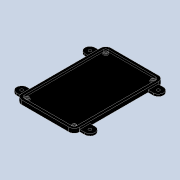
# Autodesk Inventor part: BTT Octopus 1.1 Mount
Saved by Autodesk Inventor 2022 (Build 260153000, 153)
## iProperties
Created: 2022-01-02
Part Number: BTT Octopus 1.1 Mount
Material: Generic
Document SubType Name: Modeling
Designer: Coy
Density: 1 g/cm^3
Appearance: Anodized - Black
Author: Coy
Autodesk Inventor part; units mm, degrees
ref_plane "YZ Plane" through (0, 0, 0) normal (1, 0, 0) x (0, 1, 0)
ref_plane "XZ Plane" through (0, 0, 0) normal (0, 1, 0) x (-1, 0, 0)
ref_plane "XY Plane" through (0, 0, 0) normal (0, 0, 1) x (1, 0, 0)
sketch "Sketch1" plane through (0, 0, 0) normal (0, 1, 0) x (-1, 0, 0)
  line L0 (5, 0) -> (95.5, 0)
  line L1 (100.5, 5) -> (100.5, 155.5)
  line L2 (95.5, 160.5) -> (5, 160.5)
  line L3 (0, 155.5) -> (0, 5)
  arc A0 (100.5, 155.5) -> (95.5, 160.5) centre (95.5, 155.5) ccw
  arc A1 (95.5, 0) -> (100.5, 5) centre (95.5, 5) ccw
  arc A2 (0, 5) -> (5, 0) centre (5, 5) ccw
  arc A3 (5, 160.5) -> (0, 155.5) centre (5, 155.5) ccw
  line L4 (105.5, 155.5) -> (105.5, 5)
  arc A4 (95.5, -5) -> (105.5, 5) centre (95.5, 5) ccw
  line L5 (95.5, -5) -> (5, -5)
  arc A5 (-5, 5) -> (5, -5) centre (5, 5) ccw
  line L6 (-5, 5) -> (-5, 155.5)
  arc A6 (5, 165.5) -> (-5, 155.5) centre (5, 155.5) ccw
  line L7 (5, 165.5) -> (95.5, 165.5)
  arc A7 (105.5, 155.5) -> (95.5, 165.5) centre (95.5, 155.5) ccw
  point P0 (0, 0)
  point P1 (100.5, 160.5)
  point P2 (100.5, 0)
  point P3 (0, 160.5)
  dimension "d0" = 100.5
  dimension "d1" = 160.5
  dimension "d2" = 5
  dimension "d3" = 5
  constraints: 16 end point, 16 point on circle, 8 centre point, 8 point on line, 8 tangent, 4 parallel, 3 equal radius, 2 perpendicular, 1 horizontal, 7 other
  measures "d0" distance of point (0, 160.5) point (100.5, 160.5)
  measures "d1" distance of point (100.5, 160.5) point (100.5, 0)
  measures "d2" radius of A0
  measures "d3" distance between parallel lines of L1 L4
extrude "Extrusion1" add sketch "Sketch1" along normal blind 4
sketch "Sketch2" plane through (0, 0, 0) normal (0, -1, 0) x (1, 0, 0)
  line L0 (5, 155.5) -> (5, 5) projected
  arc A0 (5, 155.5) -> (-5, 165.5) centre (-5, 155.5) ccw projected
  line L1 (-95.5, 165.5) -> (-5, 165.5) projected
  arc A1 (-95.5, 165.5) -> (-105.5, 155.5) centre (-95.5, 155.5) ccw projected
  line L2 (-105.5, 5) -> (-105.5, 155.5) projected
  arc A2 (-105.5, 5) -> (-95.5, -5) centre (-95.5, 5) ccw projected
  line L3 (-5, -5) -> (-95.5, -5) projected
  arc A3 (-5, -5) -> (5, 5) centre (-5, 5) ccw projected
  arc A4 (-5, 0) -> (0, 5) centre (-5, 5) ccw projected
  line L4 (-95.5, 0) -> (-5, 0) projected
  arc A5 (-100.5, 5) -> (-95.5, 0) centre (-95.5, 5) ccw projected
  line L5 (-100.5, 155.5) -> (-100.5, 5) projected
  arc A6 (-95.5, 160.5) -> (-100.5, 155.5) centre (-95.5, 155.5) ccw projected
  line L6 (-5, 160.5) -> (-95.5, 160.5) projected
  arc A7 (0, 155.5) -> (-5, 160.5) centre (-5, 155.5) ccw projected
  line L7 (0, 5) -> (0, 155.5) projected
  line L8 (14.75, 145.25) -> (-115.25, 145.25) construction
  line L9 (-115.25, 145.25) -> (-115.25, 15.25) construction
  line L10 (-115.25, 15.25) -> (14.75, 15.25) construction
  line L11 (14.75, 15.25) -> (14.75, 145.25) construction
  circle A8 centre (14.75, 145.25) radius 2.75
  arc A9 (14.75, 135.5) -> (14.75, 155) centre (14.75, 145.25) ccw
  line L12 (5, 155.5) -> (5, 5) projected
  line L13 (5, 155.5) -> (5, 5) projected
  line L14 (5, 135.5) -> (14.75, 135.5)
  line L15 (5, 155) -> (14.75, 155)
  line L16 (0, 5) -> (0, 155.5) construction
  line L17 (0, 80.25) -> (-100.5, 80.25) construction
  line L18 (-100.5, 155.5) -> (-100.5, 5) construction
  line L19 (-50.25, 80.25) -> (-50.25, 145.25) construction
  circle A10 centre (14.75, 15.25) radius 2.75
  arc A11 (14.75, 5.5) -> (14.75, 25) centre (14.75, 15.25) ccw
  line L20 (5, 25) -> (14.75, 25)
  line L21 (5, 5.5) -> (14.75, 5.5)
  circle A12 centre (-115.25, 145.25) radius 2.75
  arc A13 (-115.25, 155) -> (-115.25, 135.5) centre (-115.25, 145.25) ccw
  line L22 (-105.5, 135.5) -> (-115.25, 135.5)
  line L23 (-105.5, 155) -> (-115.25, 155)
  arc A14 (-115.25, 25) -> (-115.25, 5.5) centre (-115.25, 15.25) ccw
  line L24 (-105.5, 25) -> (-115.25, 25)
  circle A15 centre (-115.25, 15.25) radius 2.75
  line L25 (-105.5, 5.5) -> (-115.25, 5.5)
  point P0 (0, 0)
  dimension "d6" = 130
  dimension "d7" = 130
  dimension "d8" = 110.5
  dimension "d9" = 9.75
  dimension "d10" = 170.5
  dimension "d11" = 20.25
  dimension "d12" = 5.5
  constraints: 28 end point, 15 symmetric about line, 8 centre point, 8 point on circle, 4 midpoint, 3 perpendicular, 3 tangent, 2 parallel, 2 point on line, 1 coincident, 1 horizontal, 6 other
  measures "d6" distance of L10.end L9.end
  measures "d7" distance of L9.end L8.end
  measures "d8" distance between parallel lines of L2 L0
  measures "d9" distance between parallel lines of L0 L11
  measures "d10" distance between parallel lines of L3 L1
  measures "d11" distance between parallel lines of L1 L8
  measures "d12" diameter of A8
extrude "Extrusion2" add sketch "Sketch2" along normal blind 4 contours L0 A3 L3 A2 L2 A1 L1 A0 | L15 A9 L14 L0 | L20 A11 L21 L0 | L2 L22 A13 L23 | L2 L25 A14 L24 | L4 A5 L5 A6 L6 A7 L7 A4
sketch "Sketch3" plane through (0, 0, 0) normal (0, 1, 0) x (1, 0, 0)
  line L0 (-5.25, -155.25) -> (-95.25, -155.25) construction
  line L1 (-95.25, -155.25) -> (-95.25, -5.25) construction
  line L2 (-95.25, -5.25) -> (-5.25, -5.25) construction
  line L3 (-5.25, -5.25) -> (-5.25, -155.25) construction
  line L4 (-50.25, -155.25) -> (-50.25, -160.5) construction
  line L5 (-5, -160.5) -> (-95.5, -160.5) construction
  line L6 (-5.25, -80.25) -> (0, -80.25) construction
  line L7 (-50.25, -5.25) -> (-50.25, 0) construction
  line L8 (-95.5, 0) -> (-5, 0) construction
  line L9 (-95.25, -80.25) -> (-100.5, -80.25) construction
  line L10 (-100.5, -155.5) -> (-100.5, -5) construction
  line L11 (0, -5) -> (0, -155.5) projected
  line L12 (-100.5, -155.5) -> (-100.5, -5) projected
  arc A0 (-5, -160.5) -> (0, -155.5) centre (-5, -155.5) ccw projected
  arc A1 (-100.5, -155.5) -> (-95.5, -160.5) centre (-95.5, -155.5) ccw projected
  circle A2 centre (-5.25, -5.25) radius 3.5
  circle A3 centre (-5.25, -155.25) radius 3.5
  circle A4 centre (-95.25, -155.25) radius 3.5
  circle A5 centre (-95.25, -5.25) radius 3.5
  point P0 (0, 0)
  dimension "d15" = 90
  dimension "d16" = 150
  dimension "d17" = 7
  dimension "d18" = 7
  dimension "d19" = 7
  dimension "d20" = 7
  constraints: 16 end point, 8 midpoint, 4 centre point, 4 coincident, 4 parallel, 2 collinear, 2 horizontal, 2 perpendicular, 2 vertical
  measures "d15" distance of L1.end L2.end
  measures "d16" distance of L0.end L1.end
  measures "d17" diameter of A2
  measures "d18" diameter of A5
  measures "d19" diameter of A3
  measures "d20" diameter of A4
extrude "Extrusion3" add sketch "Sketch3" along normal blind 2.3
sketch "Sketch4" plane through (-95.25, 2.3, 155.25) normal (0, 1, 0) x (1, 0, 0)
  circle A0 centre (90, 0) radius 3.5 projected
  circle A1 centre (0, 0) radius 3.5 projected
  circle A2 centre (90, 150) radius 3.5 projected
  circle A3 centre (0, 150) radius 3.5 projected
  circle A4 centre (90, 0) radius 1.5
  circle A5 centre (0, 0) radius 3.5 projected
  circle A6 centre (0, 0) radius 1.5
  circle A7 centre (90, 150) radius 3.5 projected
  circle A8 centre (90, 150) radius 1.5
  circle A9 centre (0, 150) radius 1.5
  point P0 (95.25, 155.25)
  dimension "d23" = 3
  dimension "d24" = 3
  dimension "d25" = 3
  dimension "d26" = 3
  constraints: 4 centre point, 4 coincident
  measures "d23" diameter of A4
  measures "d24" diameter of A6
  measures "d25" diameter of A8
  measures "d26" diameter of A9
extrude "Extrusion4" cut sketch "Sketch4" against normal through all contours A4 | A6 | A8 | A9
chamfer "Chamfer1" distance 1 angle 45 4 edges at (-96.75, 2.3, 155.25) (-6.75, 2.3, 155.25) (-6.75, 2.3, 5.25) (-96.75, 2.3, 5.25)
chamfer "Chamfer2" distance 1 angle 45 4 edges at (-98.75, 0, 155.25) (-8.75, 0, 155.25) (-98.75, 0, 5.25) (-8.75, 0, 5.25)
equation "\"d9\" = -0.5 * d8 + 0.5 * d6"
equation "\"d11\" = -0.5 * d7 + 0.5 * d10"
equation "\"d18\" = d17"
equation "\"d19\" = d17"
equation "\"d20\" = d17"
equation "\"d24\" = d23"
equation "\"d25\" = d23"
equation "\"d26\" = d23"
body "Solid1"
